Autodesk Fusion 360 part; units mm, degrees
(part 3 of 3)
equation "guscio_cannone_foro_canna = 11.0 mm" comment "Passaggio canna nel guscio mobile"
named bodies: "Piano_inferiore_con_colonnine_M3", "Piano_superiore", "Guscio_laterale_continuo_166x176_Z0_Z76", "Supporto_batteria_con_apertura_cavi", "Tetto_removibile_con_supporto_stepper_e_boss_M3", "Corpo_stepper", "Piastra_adattatore_rotante", "Base_parte_fissa", "Corpo_SG90_Sinistro", "Corpo_SG90_Destro", "Barretta_Sinistra_01", "Barretta_Sinistra_02", "Barretta_Destra_01", "Barretta_Destra_02", "Piastra_culla_mobile", "PCB_modulo_cannone_50x50", "Appoggio_solenoide_su_PCB", "Corpo_solenoide_riferimento", "Canna_tubolare_esterna", "Parete_posteriore_guscio_torretta", "Parete_esterna_carter_Sinistro", "Parete_esterna_carter_Destro", "Parete_mobile_Ovest", "Canna_tubolare_esterna (1)"
